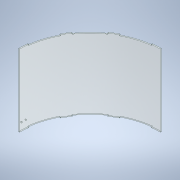
# Autodesk Inventor part: Lexan Shield
Saved by Autodesk Inventor 2020 (Build 240168000, 168)
## iProperties
Created: 2021-01-17
Part Number: Lexan Shield
Material: Glass
Document SubType Name: Modeling
Designer: magda
Density: 2.18 g/cm^3
Appearance: Clear
Author: magda
Autodesk Inventor part; units mm, degrees
ref_plane "YZ Plane" through (0, 0, 0) normal (1, 0, 0) x (0, 1, 0)
ref_plane "XZ Plane" through (0, 0, 0) normal (0, 1, 0) x (-1, 0, 0)
ref_plane "XY Plane" through (0, 0, 0) normal (0, 0, 1) x (1, 0, 0)
sketch "Sketch1" plane through (0, 0, 0) normal (0, 1, 0) x (-1, 0, 0)
  circle A0 centre (0, 0) radius 203.2
  circle A1 centre (0, 0) radius 206.375
  line L0 (0, 0) -> (206.375, 0)
  line L1 (206.375, 0) -> (206.375, -206.375)
  line L2 (206.375, -206.375) -> (0, -206.375)
  line L3 (0, -206.375) -> (0, 0)
  line L4 (0, 0) -> (232.171, 0)
  line L5 (0, 0) -> (0, -316.5803)
  line L6 (0, 0) -> (292.5853, -35.925)
  line L7 (0, 0) -> (289.4189, -151.7338)
  line L8 (0, 0) -> (278.5021, -192.6046)
  line L9 (0, 0) -> (176.5503, -255.2879)
  line L10 (0, 0) -> (153.0772, -291.9813)
  line L11 (0, 0) -> (29.3426, -238.9764)
  point P0 (0, -203.2)
  point P1 (203.2, 0)
  point P2 (201.6854, -24.7639)
  point P3 (204.8367, -25.1508)
  point P4 (167.1269, -115.5805)
  point P5 (169.7382, -117.3864)
  point P6 (182.7788, -95.8256)
  point P7 (179.9669, -94.3513)
  point P8 (94.3513, -179.9669)
  point P9 (95.8256, -182.7788)
  point P10 (117.3864, -169.7382)
  point P11 (115.5805, -167.1269)
  point P12 (25.1508, -204.8367)
  point P13 (24.7639, -201.6854)
  dimension "d0" = 406.4
  dimension "d1" = 412.75
  dimension "d12" = 7
  dimension "d13" = 27.667
  dimension "d14" = 7
  dimension "d15" = 7
  dimension "d16" = 27.667
  dimension "d17" = 7
  constraints: 24 end point, 2 centre point, 2 coincident, 2 parallel, 2 perpendicular, 2 tangent, 1 horizontal, 1 vertical
  measures "d0" diameter of A0
  measures "d1" diameter of A1
  measures "d12" angle of L6 L0
  measures "d13" angle of L7 L0
  measures "d14" angle of L8 L7
  measures "d15" angle of L3 L11
  measures "d16" angle of L5 L10
  measures "d17" angle of L10 L9
extrude "Extrusion1" add sketch "Sketch1" along normal blind 203.2 contours L0 A1 L6 A0 | A0 L11 A1 L3 | L6 A1 L7 A0 | A0 L10 A1 L11 | L7 A1 L8 A0 | L8 A1 L9 A0 | L9 A1 L10 A0
extrude "Extrusion3" add sketch "Sketch1" along normal blind 205.74 and the other way blind 2.54 contours L0 A1 L6 A0 | A0 L11 A1 L3 | L7 A1 L8 A0 | L9 A1 L10 A0
ref_plane "Work Plane1" through (-206.375, 0, 0) normal (-0.9981348, 0, -0.0610485) x (0, 1, 0)
sketch "Sketch2" plane through (-206.375, 0, 0) normal (-0.9981348, 0, -0.0610485) x (0, 1, 0)
  line L0 (0, 95.7875) -> (0, 25.004) projected
  circle A0 centre (19.05, 6.5438) radius 1.5875
  circle A1 centre (19.05, 18.654) radius 1.5875
  line L1 (-2.54, 0.1938) -> (205.74, 0.1938) projected
  line L2 (-2.54, 25.004) -> (0, 25.004) projected
  point P0 (0, 12.5989)
  dimension "d25" = 3.175
  dimension "d26" = 3.175
  dimension "d27" = 19.05
  dimension "d28" = 19.05
  dimension "d29" = 6.35
  dimension "d30" = 6.35
  constraints: 2 centre point
  measures "d25" diameter of A0
  measures "d26" diameter of A1
  measures "d27" distance from line of L0 A1.centre
  measures "d28" distance from line of L0 A0.centre
  measures "d29" distance from line of L1 A0.centre
  measures "d30" distance from line of L2 A1.centre
extrude "Extrusion4" cut sketch "Sketch2" against normal blind 205.74
body "Solid1"
